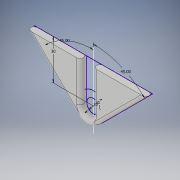
# Autodesk Inventor part: rope loop for patella
Saved by Autodesk Inventor 2019 (Build 230136000, 136)
## iProperties
Created: 2018-09-13
Part Number: rope loop for patella
Material: Generic
Document SubType Name: Modeling
Designer: HIVE
Density: 1 g/cm^3
Appearance: Default
Author: HIVE
## iProperties of the stored document rope loop for patella_3DPrint.ipt
Created: 2018-09-13
Part Number: rope loop for patella_3DPrint
Material: Generic
Document SubType Name: Modeling
Designer: HIVE
Density: 1 g/cm^3
Appearance: Default
Author: HIVE
Autodesk Inventor part; units mm, degrees
ref_plane "YZ Plane" through (0, 0, 0) normal (1, 0, 0) x (0, 1, 0)
ref_plane "XZ Plane" through (0, 0, 0) normal (0, 1, 0) x (-1, 0, 0)
ref_plane "XY Plane" through (0, 0, 0) normal (0, 0, 1) x (1, 0, 0)
sketch "Sketch1" plane through (0, 0, 0) normal (0, 0, 1) x (1, 0, 0)
  arc A0 (-5, 0) -> (5, 0) centre (0, 0) ccw
  circle A1 centre (0, 0) radius 10
  line L0 (-7.0711, -7.0711) -> (-44.1421, 30)
  line L1 (-44.1421, 30) -> (-5, 30)
  line L2 (44.1421, 30) -> (7.0711, -7.0711)
  line L3 (0, -18) -> (0, 38) projected
  line L4 (-5, 0) -> (-5, 30)
  line L5 (5, 0) -> (5, 30)
  line L6 (-5, 30) -> (5, 30)
  line L7 (5, 30) -> (44.1421, 30)
  arc A2 (0, 5) -> (-5, 0) centre (0, 0) ccw
  arc A3 (5, 0) -> (0, 5) centre (0, 0) ccw
  dimension "d0" = 10
  dimension "d1" = 20
  dimension "d2" = 45
  dimension "d3" = 45
  dimension "d4" = 30
  constraints: 14 end point, 8 point on circle, 6 perpendicular, 6 tangent, 4 centre point, 3 horizontal, 2 coincident, 2 point on line
  measures "d0" diameter of A0
  measures "d1" diameter of A1
  measures "d2" angle of L0 L3
  measures "d3" angle of L2 L3
  measures "d4" distance from line of L1 point (0, 0)
extrude "Extrusion2" add sketch "Sketch1" along normal blind 5 contours A0 L3 A1 L4 | L4 A1 L3 A2 | A0 L5 A1 L3 | L4 L6 L3 A1 | A1 L0 L1 L4 | L3 A1 L5 A3 | L3 L6 L5 A1 | L5 L7 L2 A1
extrude "Extrusion3" cut sketch "Sketch1" along normal blind 5 contours L4 A1 L3 A2 | L4 L6 L3 A1 | L3 A1 L5 A3 | L3 L6 L5 A1
fillet "Fillet1" radius 2.5 12 edges at (0, -10, 5) (25.6066, 11.4645, 5) (-25.6066, 11.4645, 5) (0, -10, 0) (25.6066, 11.4645, 0) (-25.6066, 11.4645, 0) (-5, 15, 5) (5, 15, 5) (0, -5, 5) (5, 15, 0) (-5, 15, 0) (0, -5, 0)
body "Solid2"
